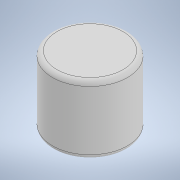
# Autodesk Inventor part: turbidity-sensor
Saved by Autodesk Inventor 2020.3 (Build 243373000, 373)
## iProperties
Created: 2021-04-12
Part Number: turbidity-sensor
Material: Generic
Document SubType Name: Modeling
Designer: Nicholas
Density: 1 g/cm^3
Appearance: Default
Author: Nicholas
Autodesk Inventor part; units mm, degrees
ref_plane "YZ Plane" through (0, 0, 0) normal (1, 0, 0) x (0, 1, 0)
ref_plane "XZ Plane" through (0, 0, 0) normal (0, 1, 0) x (-1, 0, 0)
ref_plane "XY Plane" through (0, 0, 0) normal (0, 0, 1) x (1, 0, 0)
sketch "Sketch1" plane through (0, 0, 0) normal (0, 1, 0) x (-1, 0, 0)
  circle A0 centre (0, 0) radius 16.5
  dimension "d0" = 33
  constraints: 1 centre point, 1 coincident
  measures "d0" diameter of A0
extrude "Extrusion1" add sketch "Sketch1" along normal blind 30
fillet "Fillet1" radius 2 2 edges at (16.5, 30, 0) (16.5, 0, 0)
body "Solid1"
